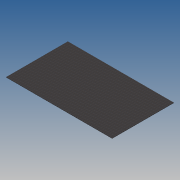
# Autodesk Inventor part: porch
Saved by Autodesk Inventor 2013 (Build 170138000, 138)
## iProperties
Created: 2013-08-10
Part Number: porch
Material: Concrete
Document SubType Name: Modeling
Designer: ddeboer
Mass: 2.47139e+06 g
Surface Area: 815056 cm^2
Volume: 1.02662e+06 cm^3
Density: 2.40731 g/cm^3
Author: ddeboer
Autodesk Inventor part; units mm, degrees
ref_plane "YZ Plane" through (0, 0, 0) normal (1, 0, 0) x (0, 1, 0)
ref_plane "XZ Plane" through (0, 0, 0) normal (0, 1, 0) x (-1, 0, 0)
ref_plane "XY Plane" through (0, 0, 0) normal (0, 0, 1) x (1, 0, 0)
sketch "Sketch1" plane through (0, 0, 0) normal (0, 1, 0) x (-1, 0, 0)
  line L0 (0, 0) -> (-8331.2, 0)
  line L1 (-8331.2, 0) -> (-8331.2, -4851.4)
  line L2 (-8331.2, -4851.4) -> (0, -4851.4)
  line L3 (0, -4851.4) -> (0, 0)
  dimension "d0" = 8331.2
  dimension "d1" = 4851.4
  constraints: 8 end point, 2 parallel, 1 horizontal, 1 perpendicular
  measures "d0" distance of L0.start L0.end
  measures "d1" distance of L2.end L0.start
extrude "Extrusion1" add sketch "Sketch1" along normal blind 25.4
sketch "Sketch2" plane through (0, 25.4, 0) normal (0, 1, 0) x (1, 0, 0)
  line L0 (8331.2, 0) -> (8331.2, 4851.4) projected
  line L1 (8331.2, 4851.4) -> (0, 4851.4) projected
  circle A0 centre (8286.75, 4806.95) radius 12.7
  circle A1 centre (5054.6, 4806.95) radius 12.7
  circle A2 centre (2438.4, 4806.95) radius 12.7
  circle A3 centre (-184.15, 4806.95) radius 12.7
  circle A4 centre (8286.75, 1130.3) radius 12.7
  circle A5 centre (5054.6, 1130.3) radius 12.7
  circle A6 centre (2438.4, 1130.3) radius 12.7
  circle A7 centre (-184.15, 1130.3) radius 12.7
  dimension "d4" = 25.4
  dimension "d5" = 44.45
  dimension "d6" = 44.45
  dimension "d7" = 25.4
  dimension "d8" = 3232.15
  dimension "d9" = 25.4
  dimension "d10" = 2616.2
  dimension "d11" = 25.4
  dimension "d12" = 2622.55
  dimension "d15" = 3676.65
  constraints: 8 centre point, 1 vertical, 8 other
  measures "d4" diameter of A0
  measures "d5" distance from line of L0 A0.centre
  measures "d6" distance from line of A0.centre L1
  measures "d7" diameter of A1
  measures "d8" distance of A1.centre A0.centre
  measures "d9" diameter of A2
  measures "d10" distance of A2.centre A1.centre
  measures "d11" diameter of A3
  measures "d12" distance of A3.centre A2.centre
  measures "d15" distance of A3.centre A7.centre
hole "Hole1" at (8286.75, 25.4, -1130.3) at (8286.75, 25.4, -4806.95) at (5054.6, 25.4, -1130.3) at (5054.6, 25.4, -4806.95) at (2438.4, 25.4, -4806.95) at (2438.4, 25.4, -1130.3) direction (0, -1, 0) diameter 25.4 depth 25.4 tip angle 118
sketch "Sketch3" plane through (0, 25.4, 0) normal (0, 1, 0) x (1, 0, 0)
  circle A0 centre (4165.6, 2425.7) radius 12.7
  dimension "d27" = 25.4
  constraints: 1 centre point
  measures "d27" diameter of A0
extrude "Extrusion2" cut sketch "Sketch3" against normal blind 1092.2
body "Solid1"
